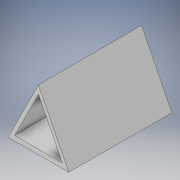
# Autodesk Inventor part: Aspax2
Saved by Autodesk Inventor 2019 (Build 230136000, 136)
## iProperties
Created: 2018-08-28
Part Number: Aspax2
Material: Genérico
Document SubType Name: Modeling
Designer: Cecilia Barrera Vill
Density: 1 g/cm^3
Appearance: Valor por defecto
Author: Cecilia Barrera Vill
Autodesk Inventor part; units mm, degrees
ref_plane "YZ Plane" through (0, 0, 0) normal (1, 0, 0) x (0, 1, 0)
ref_plane "XZ Plane" through (0, 0, 0) normal (0, 1, 0) x (-1, 0, 0)
ref_plane "XY Plane" through (0, 0, 0) normal (0, 0, 1) x (1, 0, 0)
sketch "Boceto1" plane through (0, 0, 0) normal (0, 0, 1) x (1, 0, 0)
  line L0 (0, 0) -> (50, 0)
  line L1 (50, 0) -> (50, 50)
  line L2 (50, 50) -> (0, 50)
  line L3 (0, 50) -> (0, 0)
  line L4 (0, 0) -> (25, 50)
  line L5 (50, 0) -> (25, 50)
  dimension "d0" = 50
  dimension "d1" = 50
  constraints: 12 end point, 2 parallel, 1 horizontal, 1 midpoint, 1 perpendicular
  measures "d0" distance of L2.end L1.end
  measures "d1" distance of L1.end L0.end
extrude "Extrusión1" add sketch "Boceto1" along normal blind 85 contours L4 L5 L0
sketch "Boceto2" plane through (0, 0, 85) normal (0, 0, 1) x (1, 0, 0)
  line L0 (25, 4) -> (47.7159, 4)
  line L1 (50, 0) -> (25, 50) projected
  line L2 (37.5, 25) -> (38.8416, 22.3167)
  line L3 (38.8416, 22.3167) -> (36.1584, 20.9751)
  line L4 (36.1584, 20.9751) -> (44.6459, 4)
  line L5 (25, 4) -> (2, 4)
  line L6 (25, 50) -> (0, 0) projected
  line L7 (11.1584, 22.3167) -> (13.8416, 20.9751)
  line L8 (13.8416, 20.9751) -> (5.3541, 4)
  line L9 (13.8416, 20.9751) -> (25, 43.2918)
  line L10 (25, 43.2918) -> (36.1584, 20.9751)
  dimension "d4" = 3
  dimension "d5" = 3
  dimension "d6" = 3
  constraints: 18 end point, 6 point on line, 4 perpendicular, 2 horizontal, 1 collinear, 1 midpoint
  measures "d4" distance of L2.start L2.end
  measures "d5" distance of L2.end L3.end
  measures "d6" distance of L7.start L7.end
extrude "Extrusión2" cut sketch "Boceto2" against normal blind 85 contours L5 L8 L9 L10 L4 L0
